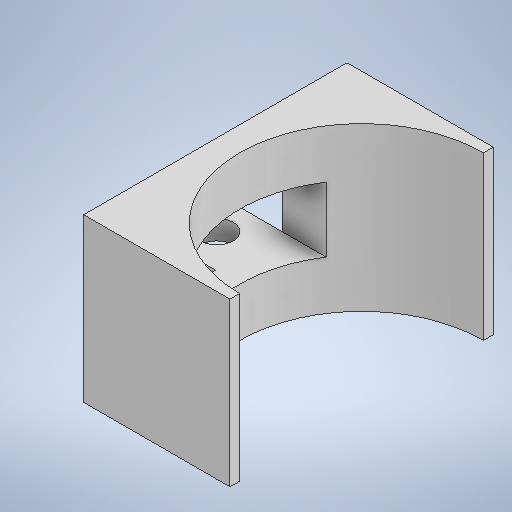
# Autodesk Inventor part: corps_pince_aimant
Saved by Autodesk Inventor 2025 (Build 290162000, 162)
## iProperties
Created: 2024-11-18
Part Number: corps_pince_aimant
Material: Générique
Document SubType Name: Modeling
Designer: chass
Density: 1 g/cm^3
Appearance: Par défaut
Author: chass
Autodesk Inventor part; units mm, degrees
ref_plane "YZ Plane" through (0, 0, 0) normal (1, 0, 0) x (0, 1, 0)
ref_plane "XZ Plane" through (0, 0, 0) normal (0, 1, 0) x (-1, 0, 0)
ref_plane "XY Plane" through (0, 0, 0) normal (0, 0, 1) x (1, 0, 0)
sketch "Esquisse2" plane through (0, 0, 0) normal (0, 1, 0) x (-1, 0, 0)
  circle A0 centre (0, 0) radius 37.5
  line L0 (45, 37.5) -> (45, -37.5)
  line L1 (45, -37.5) -> (45, -40.5)
  line L2 (45, -40.5) -> (0, -40.5)
  line L3 (0, -40.5) -> (0, -37.5)
  line L4 (0, 37.5) -> (0, 40.5)
  line L5 (0, 40.5) -> (45, 40.5)
  line L6 (45, 40.5) -> (45, 37.5)
  point P0 (22.5, 40.5)
  dimension "d0" = 75
  dimension "d4" = 81
  dimension "d13" = 45
  dimension "d14" = 45
  constraints: 14 end point, 4 perpendicular, 3 point on line, 2 point on circle, 1 centre point, 1 coincident, 1 midpoint, 1 vertical
  measures "d0" diameter of A0
  measures "d4" distance between parallel lines of L2 L5
  measures "d13" distance of L4.end L5.end
  measures "d14" distance from line of point (0, 0) L0
extrude "Extrusion1" add sketch "Esquisse2" along normal blind 50 contours A0 L4 L5 L6 L0 L1 L2 L3
sketch "Esquisse3" plane through (-45, 0, -40.5) normal (-1, 0, 0) x (0, 0, 1)
  line L0 (61, 15) -> (20, 15)
  line L1 (20, 15) -> (20, 35)
  line L2 (20, 35) -> (61, 35)
  line L3 (61, 35) -> (61, 15)
  line L4 (81, 0) -> (81, 50) projected
  line L5 (0, 0) -> (0, 50) projected
  line L6 (0, 0) -> (81, 0) projected
  line L7 (0, 50) -> (81, 50) projected
  point P0 (40.5, 0)
  point P1 (61, 25)
  dimension "d7" = 20
  dimension "d8" = 20
  dimension "d9" = 15
  dimension "d10" = 15
  constraints: 8 end point, 2 parallel, 1 horizontal, 1 midpoint, 1 perpendicular
  measures "d7" distance from line of point (61, 25) L4
  measures "d8" distance between parallel lines of L5 L1
  measures "d9" distance between parallel lines of L6 L0
  measures "d10" distance between parallel lines of L7 L2
extrude "Extrusion2" cut sketch "Esquisse3" against normal blind 50 contours L0 L1 L2 L3
sketch "Esquisse4" plane through (-45, 0, -40.5) normal (-1, 0, 0) x (0, 0, 1)
  line L0 (61, 15) -> (20, 15) projected
  line L1 (20, 15) -> (40.5, 15)
  line L2 (40.5, 15) -> (40.5, 9)
  line L3 (40.5, 9) -> (20, 9)
  line L4 (20, 9) -> (20, 15)
  point P0 (40.5, 0)
  constraints: 8 end point, 2 parallel, 1 horizontal, 1 perpendicular
extrude "Extrusion3" add sketch "Esquisse4" along normal blind 20
sketch "Esquisse5" plane through (-45, 9, -20.5) normal (0, -1, 0) x (1, 0, 0)
  circle A0 centre (-10, 10) radius 5
  point P0 (45, 20.5)
  dimension "d17" = 10
  constraints: 1 centre point
  measures "d17" diameter of A0
extrude "Extrusion4" cut sketch "Esquisse5" against normal blind 20
